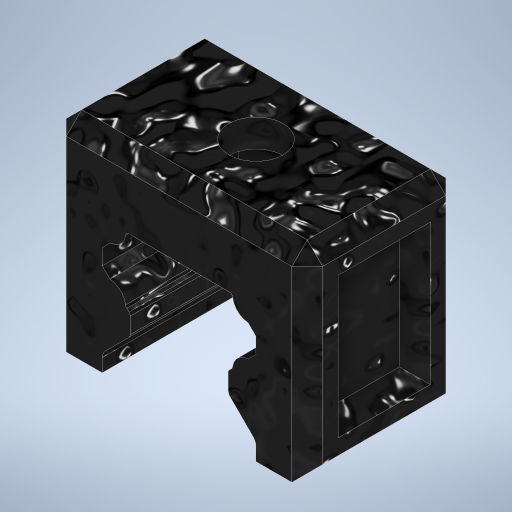
# Autodesk Inventor part: Tope Final
Saved by Autodesk Inventor 2023 (Build 270158000, 158)
## iProperties
Created: 2023-12-13
Part Number: Tope Final
Material: PET Plastic
Document SubType Name: Modeling
Designer: juanp
Density: 1.541 g/cm^3
Appearance: Black
Author: juanp
Autodesk Inventor part; units mm, degrees
ref_plane "YZ Plane" through (0, 0, 0) normal (1, 0, 0) x (0, 1, 0)
ref_plane "XZ Plane" through (0, 0, 0) normal (0, 1, 0) x (-1, 0, 0)
ref_plane "XY Plane" through (0, 0, 0) normal (0, 0, 1) x (1, 0, 0)
sketch "Sketch1" plane through (0, 0, 0) normal (0, 0, 1) x (1, 0, 0)
  arc A0 (-5.217, 1.3451) -> (-5.1032, 1.1142) centre (-4.8204, 1.397) ccw projected
  line L0 (-5.1032, 1.1142) -> (-4.8872, 0.8982) projected
  arc A1 (-4.77, 0.6153) -> (-4.8872, 0.8982) centre (-5.17, 0.6153) ccw projected
  line L1 (-4.77, 0.6153) -> (-4.77, -0.9467) projected
  arc A2 (-4.8872, -1.2296) -> (-4.77, -0.9467) centre (-5.17, -0.9467) ccw projected
  line L2 (-4.8872, -1.2296) -> (-7.2071, -3.5495) projected
  arc A3 (-7.2071, -3.5495) -> (-7.5, -4.2566) centre (-6.5, -4.2566) ccw projected
  line L3 (-7.5, -4.2566) -> (-7.5, -6.8) projected
  line L4 (-7.5, -6.8) -> (-6.8, -7.5) projected
  line L5 (-6.8, -7.5) -> (6.8, -7.5) projected
  line L6 (6.8, -7.5) -> (7.5, -6.8) projected
  line L7 (7.5, -6.8) -> (7.5, -4.2566) projected
  arc A4 (7.5, -4.2566) -> (7.2071, -3.5495) centre (6.5, -4.2566) ccw projected
  line L8 (7.2071, -3.5495) -> (4.8872, -1.2296) projected
  arc A5 (4.77, -0.9467) -> (4.8872, -1.2296) centre (5.17, -0.9467) ccw projected
  line L9 (4.77, -0.9467) -> (4.77, 0.6153) projected
  arc A6 (4.8872, 0.8982) -> (4.77, 0.6153) centre (5.17, 0.6153) ccw projected
  line L10 (4.8872, 0.8982) -> (5.1032, 1.1142) projected
  arc A7 (5.1032, 1.1142) -> (5.217, 1.3451) centre (4.8204, 1.397) ccw projected
  arc A8 (6.7419, 2.7529) -> (5.217, 1.3451) centre (6.8233, 1.1349) ccw projected
  line L11 (6.7419, 2.7529) -> (7.5, 3.511) projected
  line L12 (7.5, 3.511) -> (7.5, 5.049) projected
  line L13 (7.5, 5.049) -> (6.7304, 5.8186) projected
  arc A9 (5.2183, 7.2157) -> (6.7304, 5.8186) centre (6.8233, 7.436) ccw projected
  arc A10 (5.2183, 7.2157) -> (5.1049, 7.4441) centre (4.822, 7.1613) ccw projected
  line L14 (5.1049, 7.4441) -> (5.049, 7.5) projected
  line L15 (5.049, 7.5) -> (-5.049, 7.5) projected
  line L16 (-5.049, 7.5) -> (-5.1049, 7.4441) projected
  arc A11 (-5.1049, 7.4441) -> (-5.2183, 7.2157) centre (-4.822, 7.1613) ccw projected
  arc A12 (-6.7304, 5.8186) -> (-5.2183, 7.2157) centre (-6.8233, 7.436) ccw projected
  line L17 (-6.7304, 5.8186) -> (-7.5, 5.049) projected
  line L18 (-7.5, 5.049) -> (-7.5, 3.511) projected
  line L19 (-7.5, 3.511) -> (-6.7419, 2.7529) projected
  arc A13 (-5.217, 1.3451) -> (-6.7419, 2.7529) centre (-6.8233, 1.1349) ccw projected
  line L20 (-7.5, -5.5283) -> (-12.5, -5.5283)
  line L21 (-12.5, -5.5283) -> (-12.5, 14.2)
  line L22 (-12.5, 14.2) -> (12.5, 14.2)
  line L23 (12.5, 14.2) -> (12.5, -5.5283)
  line L24 (12.5, -5.5283) -> (7.5, -5.5283)
  point P0 (0, 0)
  dimension "d1" = 25
  dimension "d2" = 6.7
  constraints: 10 end point, 2 midpoint, 2 perpendicular, 1 collinear, 1 horizontal, 1 parallel, 1 point on line
  measures "d1" distance between parallel lines of L23 L21
  measures "d2" distance between parallel lines of L15 L22
extrude "Extrusion1" add sketch "Sketch1" against normal blind 15 contours A0 L0 A1 L1 A2 L2 A3 L3 L20 L21 L22 L23 L24 L7 A4 L8 A5 L9 A6 L10 A7 A8 L11 L12 L13 A9 A10 L14 L15 L16 A11 A12 L17 L18 L19 A13
chamfer "Chamfer1" distance 1.5 angle 45 10 edges at (-12.5, -5.5283, -7.5) (-12.5, 4.3358, -15) (-12.5, 4.3358, 0) (0, 14.2, -15) (0, 14.2, 0) (-12.5, 14.2, -7.5) (12.5, 4.3358, -15) (12.5, 4.3358, 0) (12.5, -5.5283, -7.5) (12.5, 14.2, -7.5)
sketch "Sketch2" plane through (-5.049, 7.5, 0) normal (0, -1, 0) x (1, 0, 0)
  point P0 (5.049, 0)
sketch "Sketch3" plane through (-5.049, 7.5, 0) normal (0, -1, 0) x (1, 0, 0)
  line L0 (5.049, 0) -> (5.049, -15) construction
  line L1 (10.098, -15) -> (0, -15) projected
  circle A0 centre (5.049, -7.5) radius 2.65
  dimension "d8" = 5.3
  constraints: 2 end point, 2 midpoint, 1 centre point
  measures "d8" diameter of A0
extrude "Extrusion2" cut sketch "Sketch3" against normal blind 15
sketch "Sketch4" plane through (-5.049, 7.5, 0) normal (0, -1, 0) x (1, 0, 0)
  circle A0 centre (5.049, -7.5) radius 2.65 projected
  line L0 (1.049, -5.1906) -> (5.049, -2.8812)
  line L1 (5.049, -2.8812) -> (9.049, -5.1906)
  line L2 (9.049, -5.1906) -> (9.049, -9.8094)
  line L3 (9.049, -9.8094) -> (5.049, -12.1188)
  line L4 (5.049, -12.1188) -> (1.049, -9.8094)
  line L5 (1.049, -9.8094) -> (1.049, -5.1906)
  point P0 (5.049, 0)
  dimension "d11" = 8
  constraints: 12 end point, 1 coincident, 1 vertical, 13 other
  measures "d11" distance between parallel lines of L0 L3
extrude "Extrusion3" cut sketch "Sketch4" against normal blind 4
sketch "Sketch5" plane through (12.5, -4.0283, -13.5) normal (1, 0, 0) x (0, 0, -1)
  line L0 (0, 0) -> (-12, 0) projected
  line L1 (0, 16.7283) -> (0, 0) projected
  line L2 (-12, 16.7283) -> (0, 16.7283) projected
  line L3 (-12, 0) -> (-12, 16.7283) projected
  line L4 (-10.5, 15.2283) -> (-1.5, 15.2283)
  line L5 (-1.5, 15.2283) -> (-1.5, 1.5)
  line L6 (-1.5, 1.5) -> (-10.5, 1.5)
  line L7 (-10.5, 1.5) -> (-10.5, 15.2283)
  point P0 (-13.5, 4.0283)
  dimension "d14" = 1.5
  constraints: 8 end point, 3 other
  measures "d14" distance between parallel lines of L3 L7
extrude "Extrusion4" cut sketch "Sketch5" against normal blind 1.5 contours L4 L5 L6 L7
chamfer "Chamfer2" distance 1.5 angle 45 4 edges at (11, 4.3358, -3) (11, -2.5283, -7.5) (11, 11.2, -7.5) (11, 4.3358, -12)
mirror "Mirror1" about plane through (0, 0, 0) normal (1, 0, 0) of "Extrusion4", "Chamfer2"
body "Solid1"
